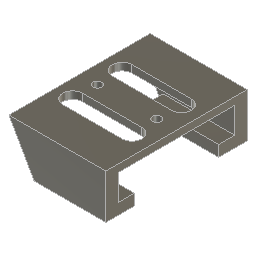
Крепление аккамулятора FengBao_ver2 (Autodesk Fusion 360 design; units mm, degrees)
Autodesk Fusion 360 part; units mm, degrees
note: some values were not read from the file. Chosen so that the rebuilt part matches the saved one: which bodies a step acts on; which face or edge a step refers to. Set by a fixed rule: which sketch regions a step uses.
sketch "Sketch1" plane through (0, 0, 0) normal (0, 0, 1) x (1, 0, 0)
  line L0 (-2, 17.05) -> (-31, 17.05)
  line L1 (-31, -17.05) -> (-2, -17.05)
  line L2 (-2, 23.55) -> (-31, 23.55)
  line L3 (-31, 28.55) -> (-31, -28.55)
  line L4 (-31, -23.55) -> (-2, -23.55)
  line L5 (-2, 28.55) -> (-31, 28.55)
  line L6 (-31, -28.55) -> (-2, -28.55)
  circle A0 centre (-34, 0) radius 1.75
  circle A1 centre (-10, 0) radius 1.75
  line L7 (-34, -14) -> (-10, -14)
  arc A2 (-10, -14) -> (-10, -6) centre (-10, -10) ccw
  line L8 (-10, -6) -> (-34, -6)
  arc A3 (-34, -6) -> (-34, -14) centre (-34, -10) ccw
  line L9 (-34, -10) -> (-10, -10) construction
  line L10 (-10, 6) -> (-34, 6)
  arc A4 (-34, 14) -> (-34, 6) centre (-34, 10) ccw
  line L11 (-34, 14) -> (-10, 14)
  arc A5 (-10, 6) -> (-10, 14) centre (-10, 10) ccw
  line L12 (-2, 28.55) -> (-2, -28.55)
  line L13 (-31, 0) -> (-41, 0)
  line L14 (-41, 0) -> (-41, 31)
  line L15 (-41, 31) -> (-41, -30)
  dimension "d2" = 34.1
  dimension "d4" = 47.1
  dimension "d12" = 3.5
  dimension "d13" = 3.5
  constraint horizontal L0
  constraint parallel L0 L1
  constraint horizontal L2
  constraint perpendicular L2 L3
  constraint parallel L2 L4
  constraint coincident L2.end L3
  constraint coincident L4.start L3
  constraint tangent L7 A2
  constraint tangent A2 L8
  constraint parallel L7 L8
  constraint tangent L8 A3
  constraint tangent L7 A3
  constraint horizontal L9
  constraint perpendicular L6 L12
  constraint coincident L12 L4.end
  constraint coincident L12 L1.end
  constraint coincident L12 L0.start
  constraint coincident L12 L2.start
  constraint midpoint L3 L13.start
  constraint perpendicular L3 L13
  constraint perpendicular L13 L14
  constraint perpendicular L13 L15
  constraint coincident A0.centre L13
  measures "d2" distance of L0.end L1.start
  measures "d4" distance of L2.end L4.start
  measures "d12" diameter of A0
  measures "d13" diameter of A1
extrude "Extrude1" add sketch "Sketch1" along normal blind 4.5 contours L0 L2 L3 L12 | L2 L3 L5 L12 | L1 L3 L4 L12 makes body 1 at (-11.6667, -21.3833, 0) makes body 2 at (-11.6667, 20.8833, 0)
extrude "Extrude2" add sketch "Sketch1" along normal blind 15 contours L2 L3 L5 L12 | L3 L4 L6 L12 bodies 1 2
extrude "Extrude5" add sketch "Sketch1" along normal blind 18 and the other way blind -15 contours L0 L1 L3 L7 A2 L8 L10 L11 A5 L12 | L0 L2 L3 L12 | L2 L3 L5 L12 | L1 L3 L4 L12 | L3 L10 L11 A5 | L3 L4 L6 L12 | L3 L7 A2 L8 | A1 bodies 1 2
sketch "Sketch2" plane through (0, -28.55, 0) normal (0, -1, 0) x (1, 0, 0)
  line L0 (-31, 0) -> (-2, 0)
  line L1 (-2, 0) -> (-2, 18)
  line L2 (-31, 18) -> (-31, 0)
  line L3 (-31, 0) -> (-31, 8.8)
  line L4 (-31, 8.8) -> (-36, 8.8)
  line L5 (-31, 0) -> (-41.2273, 18)
  line L6 (-31, 18) -> (-41.2273, 18)
  line L7 (-2, 18) -> (-31, 18)
  line L8 (-31, 18) -> (-31, 15)
  line L9 (-31, 15) -> (-39.5227, 15)
  dimension "d14" = 8.8
  dimension "d15" = 5
  constraint coincident L0.start L2.end
  constraint perpendicular L0 L3
  constraint perpendicular L2 L4
  constraint coincident L4.end L5
  constraint coincident L2.start L6.start
  constraint perpendicular L2 L6
  constraint coincident L2 L8.end
  constraint coincident L5 L9.end
  constraint perpendicular L8 L9
  measures "d14" distance of L0.start L3.end
  measures "d15" distance of L3.end L4.end
extrude "Extrude3" add sketch "Sketch2" against normal blind 5 contours L2 L3 L4 L5 | L2 L4 L5 L9 | L2 L5 L6 L8 L9 bodies 1
extrude "Extrude4" add sketch "Sketch2" along normal blind -57.1 and the other way blind 52.1 contours L2 L3 L4 L5 | L2 L4 L5 L9 | L2 L5 L6 L8 L9 bodies 1
extrude "Extrude6" add sketch "Sketch2" against normal blind 52.1 contours L2 L5 L6 L8 L9 bodies 1
extrude "Extrude7" cut sketch "Sketch1" along normal blind 23 contours L3 L10 L11 A5 | L3 L10 A4 L11 | L3 L7 L8 A3 | L3 L7 A2 L8 | A0 L13 | A0 L13 | A1 bodies 1
